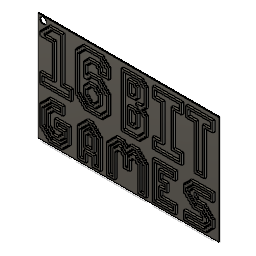
16 Bit Logo v8 (Autodesk Fusion 360 design; units mm, degrees)
Autodesk Fusion 360 part; units mm, degrees
(part 1 of 2)
sketch "Sketch1" plane through (0, 0, 0) normal (0, 0, 1) x (1, 0, 0)
  line L0 (0, 48) -> (4, 48)
  line L1 (4, 48) -> (4, 47)
  line L2 (4, 47) -> (3, 47)
  line L3 (3, 47) -> (3, 46)
  line L4 (3, 46) -> (2, 46)
  line L5 (2, 46) -> (2, 45)
  line L6 (2, 45) -> (1, 45)
  line L7 (1, 45) -> (1, 44)
  line L8 (1, 44) -> (0, 44)
  line L9 (0, 44) -> (0, 42)
  line L10 (0, 42) -> (6, 42)
  line L11 (6, 42) -> (6, 27)
  line L12 (6, 27) -> (0, 27)
  line L13 (0, 27) -> (0, 26.9)
  line L14 (0, 27) -> (0, 22)
  line L15 (7, 42) -> (7, 27)
  line L16 (7, 27) -> (7, 26)
  line L17 (7, 26) -> (1, 26)
  line L18 (0, 22) -> (15, 22)
  line L19 (15, 22) -> (15, 27)
  line L20 (15, 27) -> (11, 27)
  line L21 (11, 27) -> (11, 48)
  line L22 (1, 26) -> (1, 23)
  line L23 (1, 23) -> (14, 23)
  line L24 (14, 23) -> (14, 26)
  line L25 (14, 26) -> (10, 26)
  line L26 (10, 26) -> (10, 47)
  line L27 (10, 47) -> (5, 47)
  line L28 (5, 47) -> (5, 46)
  line L29 (5, 46) -> (4, 46)
  line L30 (4, 46) -> (4, 45)
  line L31 (4, 45) -> (3, 45)
  line L32 (3, 45) -> (3, 44)
  line L33 (3, 44) -> (2, 44)
  line L34 (2, 44) -> (2, 43)
  line L35 (2, 43) -> (6, 43)
  line L36 (7, 42) -> (7, 43)
  line L37 (7, 43) -> (6, 43)
  line L38 (17, 27) -> (17, 26)
  line L39 (17, 26) -> (18, 26)
  line L40 (18, 26) -> (18, 25)
  line L41 (18, 25) -> (19, 25)
  line L42 (19, 25) -> (19, 24)
  line L43 (19, 24) -> (20, 24)
  line L44 (20, 24) -> (20, 23)
  line L45 (20, 23) -> (21, 23)
  line L46 (21, 23) -> (21, 22)
  line L47 (21, 22) -> (30, 22)
  line L48 (30, 22) -> (30, 23)
  line L49 (30, 23) -> (31, 23)
  line L50 (31, 23) -> (31, 24)
  line L51 (31, 24) -> (32, 24)
  line L52 (32, 24) -> (32, 25)
  line L53 (32, 25) -> (33, 25)
  line L54 (33, 25) -> (33, 34)
  line L55 (33, 34) -> (32, 34)
  line L56 (32, 34) -> (32, 35)
  line L57 (32, 35) -> (31, 35)
  line L58 (31, 35) -> (31, 36)
  line L59 (31, 36) -> (30, 36)
  line L60 (30, 36) -> (30, 37)
  line L61 (30, 37) -> (29, 37)
  line L62 (29, 37) -> (29, 38)
  line L63 (29, 38) -> (23, 38)
  line L64 (23, 38) -> (23, 37)
  line L65 (23, 37) -> (22, 37)
  line L66 (22, 37) -> (22, 41)
  line L67 (22, 41) -> (23, 41)
  line L68 (23, 41) -> (23, 42)
  line L69 (23, 42) -> (24, 42)
  line L70 (24, 42) -> (24, 43)
  line L71 (24, 43) -> (27, 43)
  line L72 (27, 43) -> (27, 42)
  line L73 (27, 42) -> (28, 42)
  line L74 (28, 42) -> (28, 41)
  line L75 (28, 41) -> (28, 40)
  line L76 (28, 40) -> (33, 40)
  line L77 (33, 40) -> (33, 45)
  line L78 (33, 45) -> (32, 45)
  line L79 (32, 45) -> (32, 46)
  line L80 (32, 46) -> (31, 46)
  line L81 (31, 46) -> (31, 47)
  line L82 (31, 47) -> (30, 47)
  line L83 (30, 47) -> (30, 48)
  line L84 (17, 27) -> (17, 45)
  line L85 (17, 45) -> (18, 45)
  line L86 (18, 45) -> (18, 46)
  line L87 (18, 46) -> (19, 46)
  line L88 (19, 46) -> (19, 47)
  line L89 (19, 47) -> (20, 47)
  line L90 (20, 47) -> (20, 48)
  line L91 (29, 41) -> (32, 41)
  line L92 (32, 41) -> (32, 44)
  line L93 (32, 44) -> (31, 44)
  line L94 (31, 44) -> (31, 45)
  line L95 (31, 45) -> (30, 45)
  line L96 (30, 45) -> (30, 46)
  line L97 (30, 46) -> (29, 46)
  line L98 (29, 46) -> (29, 47)
  line L99 (29, 47) -> (21, 47)
  line L100 (21, 47) -> (21, 46)
  line L101 (21, 46) -> (20, 46)
  line L102 (20, 46) -> (20, 45)
  line L103 (20, 45) -> (19, 45)
  line L104 (19, 45) -> (19, 44)
  line L105 (19, 44) -> (18, 44)
  line L106 (18, 44) -> (18, 27)
  line L107 (18, 27) -> (19, 27)
  line L108 (19, 27) -> (19, 26)
  line L109 (19, 26) -> (20, 26)
  line L110 (20, 26) -> (20, 25)
  line L111 (20, 25) -> (21, 25)
  line L112 (21, 25) -> (21, 24)
  line L113 (21, 24) -> (22, 24)
  line L114 (22, 24) -> (22, 23)
  line L115 (22, 23) -> (29, 23)
  line L116 (29, 23) -> (29, 24)
  line L117 (29, 24) -> (29, 23)
  line L118 (29, 24) -> (30, 24)
  line L119 (30, 24) -> (30, 25)
  line L120 (30, 25) -> (31, 25)
  line L121 (31, 25) -> (31, 26)
  line L122 (31, 26) -> (32, 26)
  line L123 (32, 26) -> (32, 33)
  line L124 (32, 33) -> (31, 33)
  line L125 (31, 33) -> (31, 34)
  line L126 (31, 34) -> (30, 34)
  line L127 (30, 34) -> (30, 35)
  line L128 (30, 35) -> (29, 35)
  line L129 (29, 35) -> (30, 35)
  line L130 (29, 35) -> (29, 36)
  line L131 (29, 36) -> (28, 36)
  line L132 (28, 36) -> (28, 37)
  line L133 (28, 37) -> (24, 37)
  line L134 (24, 37) -> (24, 36)
  line L135 (24, 36) -> (23, 36)
  line L136 (23, 36) -> (23, 35)
  line L137 (23, 35) -> (21, 35)
  line L138 (21, 35) -> (21, 42)
  line L139 (21, 42) -> (22, 42)
  line L140 (22, 42) -> (22, 43)
  line L141 (22, 43) -> (23, 43)
  line L142 (23, 43) -> (23, 44)
  line L143 (23, 44) -> (28, 44)
  line L144 (28, 44) -> (28, 43)
  line L145 (28, 43) -> (29, 43)
  line L146 (29, 41) -> (29, 43)
  line L147 (23, 34) -> (27, 34)
  line L148 (27, 34) -> (27, 33)
  line L149 (27, 33) -> (28, 33)
  line L150 (28, 33) -> (28, 32)
  line L151 (28, 32) -> (29, 32)
  line L152 (29, 32) -> (28, 32)
  line L153 (29, 32) -> (29, 27)
  line L154 (29, 27) -> (28, 27)
  line L155 (28, 27) -> (28, 26)
  line L156 (28, 26) -> (27, 26)
  line L157 (27, 26) -> (27, 25)
  line L158 (27, 25) -> (23, 25)
  line L159 (23, 25) -> (23, 26)
  line L160 (23, 26) -> (23, 25)
  line L161 (23, 26) -> (22, 26)
  line L162 (22, 26) -> (22, 27)
  line L163 (22, 27) -> (21, 27)
  line L164 (21, 27) -> (21, 32)
  line L165 (21, 32) -> (22, 32)
  line L166 (22, 32) -> (22, 33)
  line L167 (22, 33) -> (23, 33)
  line L168 (23, 33) -> (23, 34)
  line L169 (23, 32) -> (24, 32)
  line L170 (24, 32) -> (24, 33)
  line L171 (24, 33) -> (26, 33)
  line L172 (26, 33) -> (26, 32)
  line L173 (26, 32) -> (27, 32)
  line L174 (27, 32) -> (27, 31)
  line L175 (27, 31) -> (28, 31)
  line L176 (28, 31) -> (28, 28)
  line L177 (28, 28) -> (27, 28)
  line L178 (27, 28) -> (27, 27)
  line L179 (27, 27) -> (26, 27)
  line L180 (26, 27) -> (26, 26)
  line L181 (24, 26) -> (26, 26)
  line L182 (24, 26) -> (24, 27)
  line L183 (24, 27) -> (23, 27)
  line L184 (23, 27) -> (23, 28)
  line L185 (23, 28) -> (22, 28)
  line L186 (22, 28) -> (22, 31)
  line L187 (22, 31) -> (23, 31)
  line L188 (23, 31) -> (22, 31)
  line L189 (23, 31) -> (23, 32)
  line L190 (30, 48) -> (39, 48)
  line L191 (39, 48) -> (39, 22)
  line L192 (39, 22) -> (48, 22)
  line L193 (48, 22) -> (48, 23)
  line L194 (48, 23) -> (49, 23)
  line L195 (49, 23) -> (49, 24)
  line L196 (49, 24) -> (50, 24)
  line L197 (50, 24) -> (50, 25)
  line L198 (50, 25) -> (51, 25)
  line L199 (51, 25) -> (51, 34)
  line L200 (51, 34) -> (50, 34)
  line L201 (50, 34) -> (50, 35)
  line L202 (50, 35) -> (49, 35)
  line L203 (49, 35) -> (49, 36)
  line L204 (49, 36) -> (50, 36)
  line L205 (50, 36) -> (50, 37)
  line L206 (50, 37) -> (51, 37)
  line L207 (51, 37) -> (51, 46)
  line L208 (51, 46) -> (50, 46)
  line L209 (50, 46) -> (50, 47)
  line L210 (50, 47) -> (49, 47)
  line L211 (49, 47) -> (49, 48)
  line L212 (40, 23) -> (40, 47)
  line L213 (40, 47) -> (48, 47)
  line L214 (48, 47) -> (48, 46)
  line L215 (48, 46) -> (49, 46)
  line L216 (49, 46) -> (49, 45)
  line L217 (49, 45) -> (50, 45)
  line L218 (50, 45) -> (50, 38)
  line L219 (50, 38) -> (49, 38)
  line L220 (49, 38) -> (49, 37)
  line L221 (49, 37) -> (46, 37)
  line L222 (46, 37) -> (46, 36)
  line L223 (46, 36) -> (47, 36)
  line L224 (47, 36) -> (47, 35)
  line L225 (47, 35) -> (48, 35)
  line L226 (48, 35) -> (48, 34)
  line L227 (48, 34) -> (49, 34)
  line L228 (49, 34) -> (49, 33)
  line L229 (49, 33) -> (50, 33)
  line L230 (50, 26) -> (50, 33)
  line L231 (50, 26) -> (49, 26)
  line L232 (49, 26) -> (49, 25)
  line L233 (49, 25) -> (48, 25)
  line L234 (48, 25) -> (48, 24)
  line L235 (48, 24) -> (47, 24)
  line L236 (47, 24) -> (47, 23)
  line L237 (47, 23) -> (40, 23)
  line L238 (46, 26) -> (46, 27)
  line L239 (46, 27) -> (47, 27)
  line L240 (47, 27) -> (47, 33)
  line L241 (47, 33) -> (46, 33)
  line L242 (46, 33) -> (46, 34)
  line L243 (46, 34) -> (42, 34)
  line L244 (42, 34) -> (42, 26)
  line L245 (42, 26) -> (46, 26)
  line L246 (43, 27) -> (43, 33)
  line L247 (43, 33) -> (45, 33)
  line L248 (45, 33) -> (45, 32)
  line L249 (45, 32) -> (46, 32)
  line L250 (46, 32) -> (46, 28)
  line L251 (46, 28) -> (45, 28)
  line L252 (45, 28) -> (45, 27)
  line L253 (43, 27) -> (45, 27)
  line L254 (42, 39) -> (42, 45)
  line L255 (42, 45) -> (46, 45)
  line L256 (46, 45) -> (46, 44)
  line L257 (46, 44) -> (47, 44)
  line L258 (47, 44) -> (47, 39)
  line L259 (47, 39) -> (46, 39)
  line L260 (46, 39) -> (46, 38)
  line L261 (46, 38) -> (42, 38)
  line L262 (42, 38) -> (42, 39)
  line L263 (43, 39) -> (43, 44)
  line L264 (45, 44) -> (43, 44)
  line L265 (45, 44) -> (45, 43)
  line L266 (45, 43) -> (46, 43)
  line L267 (46, 43) -> (46, 40)
  line L268 (46, 40) -> (45, 40)
  line L269 (45, 40) -> (45, 39)
  line L270 (43, 39) -> (45, 39)
  line L271 (49, 48) -> (54, 48)
  line L272 (54, 48) -> (54, 43)
  line L273 (54, 22) -> (54, 27)
  line L274 (54, 27) -> (58, 27)
  line L275 (58, 27) -> (58, 43)
  line L276 (58, 43) -> (54, 43)
  line L277 (54, 22) -> (68, 22)
  line L278 (68, 22) -> (68, 27)
  line L279 (68, 27) -> (64, 27)
  line L280 (64, 27) -> (64, 43)
  line L281 (64, 43) -> (68, 43)
  line L282 (68, 43) -> (68, 48)
  line L283 (55, 47) -> (55, 44)
  line L284 (55, 44) -> (59, 44)
  line L285 (59, 44) -> (59, 26)
  line L286 (59, 26) -> (55, 26)
  line L287 (55, 26) -> (55, 23)
  line L288 (55, 23) -> (67, 23)
  line L289 (67, 23) -> (67, 26)
  line L290 (67, 26) -> (63, 26)
  line L291 (63, 26) -> (63, 44)
  line L292 (63, 44) -> (67, 44)
  line L293 (67, 44) -> (67, 47)
  line L294 (67, 47) -> (55, 47)
  line L295 (70, 43) -> (70, 48)
  line L296 (70, 43) -> (74, 43)
  line L297 (74, 43) -> (74, 22)
  line L298 (74, 22) -> (79, 22)
  line L299 (79, 22) -> (79, 43)
  line L300 (79, 43) -> (82, 43)
  line L301 (82, 43) -> (83, 43)
  line L302 (83, 43) -> (83, 48)
  line L303 (83, 48) -> (82, 48)
  line L304 (71, 47) -> (82, 47)
  line L305 (82, 47) -> (82, 44)
  line L306 (82, 44) -> (78, 44)
  line L307 (78, 44) -> (78, 23)
  line L308 (78, 23) -> (75, 23)
  line L309 (75, 23) -> (78, 23)
  line L310 (75, 23) -> (75, 44)
  line L311 (75, 44) -> (71, 44)
  line L312 (71, 44) -> (71, 47)
  line L313 (0, 0) -> (83, 0)
  line L314 (83, 0) -> (83, 48)
  line L315 (83, 48) -> (0, 48)
  line L316 (0, 48) -> (0, 0)
  line L317 (0, 0) -> (0, 1)
  line L318 (0, 0) -> (0, 4)
  line L319 (0, 4) -> (1, 4)
  line L320 (1, 4) -> (1, 3)
  line L321 (1, 3) -> (2, 3)
  line L322 (2, 3) -> (2, 2)
  line L323 (2, 2) -> (3, 2)
  line L324 (3, 2) -> (3, 1)
  line L325 (3, 1) -> (4, 1)
  line L326 (4, 1) -> (4, 0)
  line L327 (4, 0) -> (11, 0)
  line L328 (4, 0) -> (11, 0)
  line L329 (11, 0) -> (11, 1)
  line L330 (11, 1) -> (12, 1)
  line L331 (12, 1) -> (12, 2)
  line L332 (12, 2) -> (13, 2)
  line L333 (13, 2) -> (13, 3)
  line L334 (13, 3) -> (14, 3)
  line L335 (14, 3) -> (14, 11)
  line L336 (14, 11) -> (7, 11)
  line L337 (7, 11) -> (7, 7)
  line L338 (7, 7) -> (11, 7)
  line L339 (11, 7) -> (11, 6)
  line L340 (11, 6) -> (10, 6)
  line L341 (10, 6) -> (10, 5)
  line L342 (10, 5) -> (9, 5)
  line L343 (9, 5) -> (9, 4)
  line L344 (9, 4) -> (6, 4)
  line L345 (6, 4) -> (6, 5)
  line L346 (6, 5) -> (5, 5)
  line L347 (5, 5) -> (5, 6)
  line L348 (5, 6) -> (4, 6)
  line L349 (4, 6) -> (4, 12)
  line L350 (4, 12) -> (5, 12)
  line L351 (5, 12) -> (5, 13)
  line L352 (5, 13) -> (6, 13)
  line L353 (6, 13) -> (6, 14)
  line L354 (6, 14) -> (11, 14)
  line L355 (11, 14) -> (11, 18)
  line L356 (11, 18) -> (4, 18)
  line L357 (4, 18) -> (4, 17)
  line L358 (4, 17) -> (3, 17)
  line L359 (3, 17) -> (3, 16)
  line L360 (3, 16) -> (2, 16)
  line L361 (2, 16) -> (2, 15)
  line L362 (2, 15) -> (1, 15)
  line L363 (1, 15) -> (1, 14)
  line L364 (1, 14) -> (0, 14)
  line L365 (1, 13) -> (1, 5)
  line L366 (1, 5) -> (2, 5)
  line L367 (2, 5) -> (2, 4)
  line L368 (2, 4) -> (3, 4)
  line L369 (3, 4) -> (3, 3)
  line L370 (3, 3) -> (4, 3)
  line L371 (4, 3) -> (4, 2)
  line L372 (4, 2) -> (5, 2)
  line L373 (5, 2) -> (5, 1)
  line L374 (5, 1) -> (10, 1)
  line L375 (10, 1) -> (10, 2)
  line L376 (10, 2) -> (11, 2)
  line L377 (11, 2) -> (11, 3)
  line L378 (11, 3) -> (12, 3)
  line L379 (12, 3) -> (12, 4)
  line L380 (12, 4) -> (13, 4)
  line L381 (13, 4) -> (13, 10)
  line L382 (13, 10) -> (8, 10)
  line L383 (8, 10) -> (8, 8)
  line L384 (8, 8) -> (12, 8)
  line L385 (12, 8) -> (12, 5)
  line L386 (12, 5) -> (11, 5)
  line L387 (11, 5) -> (11, 4)
  line L388 (11, 4) -> (10, 4)
  line L389 (10, 4) -> (10, 3)
  line L390 (10, 3) -> (5, 3)
  line L391 (5, 3) -> (5, 4)
  line L392 (5, 4) -> (4, 4)
  line L393 (4, 4) -> (4, 5)
  line L394 (4, 5) -> (3, 5)
  line L395 (3, 5) -> (3, 13)
  line L396 (3, 13) -> (4, 13)
  line L397 (4, 13) -> (4, 14)
  line L398 (4, 14) -> (5, 14)
  line L399 (5, 14) -> (5, 15)
  line L400 (5, 15) -> (10, 15)
  line L401 (10, 15) -> (10, 17)
  line L402 (10, 17) -> (5, 17)
  line L403 (5, 17) -> (5, 16)
  line L404 (5, 16) -> (4, 16)
  line L405 (4, 16) -> (4, 15)
  line L406 (4, 15) -> (3, 15)
  line L407 (3, 15) -> (3, 14)
  line L408 (3, 14) -> (2, 14)
  line L409 (2, 14) -> (2, 13)
  line L410 (2, 13) -> (1, 13)
  line L411 (11, 0) -> (12, 0)
  line L412 (11, 0) -> (18, 0)
  line L413 (18, 0) -> (18, 14)
  line L414 (18, 14) -> (19, 14)
  line L415 (19, 14) -> (19, 15)
  line L416 (19, 15) -> (20, 15)
  line L417 (20, 15) -> (20, 16)
  line L418 (20, 16) -> (21, 16)
  line L419 (21, 16) -> (21, 17)
  line L420 (21, 17) -> (22, 17)
  line L421 (22, 17) -> (22, 18)
  line L422 (22, 18) -> (25, 18)
  line L423 (25, 18) -> (25, 17)
  line L424 (25, 17) -> (26, 17)
  line L425 (26, 17) -> (26, 16)
  line L426 (26, 16) -> (27, 16)
  line L427 (27, 16) -> (27, 15)
  line L428 (27, 15) -> (28, 15)
  line L429 (28, 15) -> (28, 14)
  line L430 (28, 14) -> (29, 14)
  line L431 (29, 14) -> (29, 0)
  line L432 (28, 1) -> (28, 13)
  line L433 (28, 13) -> (27, 13)
  line L434 (27, 13) -> (27, 14)
  line L435 (27, 14) -> (26, 14)
  line L436 (26, 14) -> (26, 15)
  line L437 (26, 15) -> (25, 15)
  line L438 (25, 15) -> (25, 16)
  line L439 (25, 16) -> (24, 16)
  line L440 (24, 16) -> (24, 17)
  line L441 (24, 17) -> (23, 17)
  line L442 (23, 17) -> (23, 16)
  line L443 (23, 16) -> (22, 16)
  line L444 (22, 16) -> (22, 15)
  line L445 (22, 15) -> (21, 15)
  line L446 (21, 15) -> (21, 14)
  line L447 (21, 14) -> (20, 14)
  line L448 (20, 14) -> (20, 13)
  line L449 (20, 13) -> (19, 13)
  line L450 (28, 1) -> (26, 1)
  line L451 (19, 1) -> (21, 1)
  line L452 (19, 13) -> (19, 1)
  line L453 (22, 0) -> (22, 4)
  line L454 (22, 4) -> (25, 4)
  line L455 (25, 4) -> (25, 0)
  line L456 (25, 5) -> (22, 5)
  line L457 (22, 5) -> (21, 5)
  line L458 (25, 5) -> (26, 5)
  line L459 (26, 1) -> (26, 5)
  line L460 (21, 5) -> (21, 1)
  line L461 (21, 6) -> (26, 6)
  line L462 (26, 6) -> (26, 13)
  line L463 (26, 13) -> (25, 13)
  line L464 (25, 13) -> (25, 14)
  line L465 (25, 14) -> (24, 14)
  line L466 (24, 14) -> (24, 15)
  line L467 (24, 15) -> (23, 15)
  line L468 (23, 15) -> (23, 14)
  line L469 (23, 14) -> (22, 14)
  line L470 (22, 14) -> (22, 13)
  line L471 (22, 13) -> (21, 13)
  line L472 (21, 13) -> (21, 6)
  line L473 (29, 0) -> (32, 0)
  line L474 (32, 0) -> (32, 14)
  line L475 (32, 14) -> (33, 14)
  line L476 (33, 14) -> (33, 15)
  line L477 (33, 15) -> (34, 15)
  line L478 (34, 15) -> (34, 16)
  line L479 (34, 16) -> (35, 16)
  line L480 (35, 16) -> (35, 17)
  line L481 (35, 17) -> (36, 17)
  line L482 (36, 17) -> (36, 18)
  line L483 (36, 18) -> (40, 18)
  line L484 (40, 18) -> (40, 17)
  line L485 (40, 17) -> (41, 17)
  line L486 (41, 17) -> (41, 16)
  line L487 (41, 16) -> (42, 16)
  line L488 (42, 16) -> (42, 17)
  line L489 (42, 17) -> (43, 17)
  line L490 (43, 17) -> (43, 18)
  line L491 (43, 18) -> (47, 18)
  line L492 (47, 18) -> (47, 17)
  line L493 (47, 17) -> (48, 17)
  line L494 (48, 17) -> (48, 16)
  line L495 (48, 16) -> (49, 16)
  line L496 (49, 16) -> (49, 15)
  line L497 (49, 15) -> (50, 15)
  line L498 (50, 15) -> (50, 14)
  line L499 (50, 14) -> (51, 14)
  line L500 (51, 14) -> (51, 0)
  line L501 (50, 1) -> (50, 13)
  line L502 (50, 13) -> (49, 13)
  line L503 (49, 13) -> (49, 14)
  line L504 (49, 14) -> (48, 14)
  line L505 (48, 14) -> (48, 15)
  line L506 (48, 15) -> (47, 15)
  line L507 (47, 15) -> (47, 16)
  line L508 (47, 16) -> (46, 16)
  line L509 (46, 16) -> (46, 17)
  line L510 (46, 17) -> (44, 17)
  line L511 (44, 17) -> (44, 16)
  line L512 (44, 16) -> (43, 16)
  line L513 (43, 16) -> (43, 15)
  line L514 (43, 15) -> (42, 15)
  line L515 (42, 15) -> (42, 14)
  line L516 (42, 14) -> (41, 14)
  line L517 (41, 14) -> (41, 15)
  line L518 (41, 15) -> (40, 15)
  line L519 (40, 15) -> (40, 16)
  line L520 (40, 16) -> (39, 16)
  line L521 (39, 16) -> (39, 17)
  line L522 (39, 17) -> (37, 17)
  line L523 (37, 17) -> (37, 16)
  line L524 (37, 16) -> (36, 16)
  line L525 (36, 16) -> (36, 15)
  line L526 (36, 15) -> (35, 15)
  line L527 (35, 15) -> (35, 14)
  line L528 (35, 14) -> (34, 14)
  line L529 (34, 14) -> (34, 13)
  line L530 (34, 13) -> (33, 13)
  line L531 (33, 13) -> (33, 1)
  line L532 (33, 1) -> (35, 1)
  line L533 (35, 1) -> (35, 13)
  line L534 (35, 13) -> (36, 13)
  line L535 (36, 13) -> (36, 14)
  line L536 (36, 14) -> (37, 14)
  line L537 (37, 14) -> (37, 15)
  line L538 (37, 15) -> (39, 15)
  line L539 (39, 15) -> (39, 14)
  line L540 (39, 14) -> (40, 14)
  line L541 (40, 14) -> (40, 13)
  line L542 (40, 13) -> (41, 13)
  line L543 (41, 13) -> (41, 8)
  line L544 (41, 8) -> (42, 8)
  line L545 (42, 8) -> (42, 13)
  line L546 (42, 13) -> (43, 13)
  line L547 (43, 13) -> (43, 14)
  line L548 (43, 14) -> (44, 14)
  line L549 (44, 14) -> (44, 15)
  line L550 (44, 15) -> (46, 15)
  line L551 (46, 15) -> (46, 14)
  line L552 (46, 14) -> (47, 14)
  line L553 (47, 14) -> (47, 13)
  line L554 (47, 13) -> (48, 13)
  line L555 (48, 13) -> (48, 1)
  line L556 (48, 1) -> (50, 1)
  line L557 (47, 0) -> (47, 12)
  line L558 (47, 12) -> (46, 12)
  line L559 (46, 12) -> (46, 13)
  line L560 (46, 13) -> (44, 13)
  line L561 (44, 13) -> (44, 12)
  line L562 (44, 12) -> (43, 12)
  line L563 (43, 12) -> (43, 7)
  line L564 (43, 7) -> (40, 7)
  line L565 (40, 7) -> (40, 12)
  line L566 (40, 12) -> (39, 12)
  line L567 (39, 12) -> (39, 13)
  line L568 (39, 13) -> (37, 13)
  line L569 (37, 13) -> (37, 12)
  line L570 (37, 12) -> (36, 12)
  line L571 (36, 12) -> (36, 0)
  line L572 (51, 0) -> (54, 0)
  line L573 (54, 0) -> (54, 18)
  line L574 (54, 18) -> (65, 18)
  line L575 (65, 18) -> (65, 14)
  line L576 (65, 14) -> (58, 14)
  line L577 (58, 14) -> (58, 11)
  line L578 (58, 11) -> (61, 11)
  line L579 (61, 11) -> (61, 7)
  line L580 (61, 7) -> (58, 7)
  line L581 (58, 7) -> (58, 4)
  line L582 (58, 4) -> (65, 4)
  line L583 (65, 4) -> (65, 0)
  line L584 (64, 1) -> (64, 3)
  line L585 (64, 3) -> (57, 3)
  line L586 (57, 3) -> (57, 8)
  line L587 (57, 8) -> (60, 8)
  line L588 (60, 8) -> (60, 10)
  line L589 (60, 10) -> (57, 10)
  line L590 (57, 10) -> (57, 15)
  line L591 (57, 15) -> (64, 15)
  line L592 (64, 15) -> (64, 17)
  line L593 (64, 17) -> (55, 17)
  line L594 (55, 17) -> (55, 1)
  line L595 (55, 1) -> (64, 1)
  line L596 (65, 0) -> (69, 0)
  line L597 (69, 4) -> (69, 0)
  line L598 (69, 4) -> (78, 4)
  line L599 (78, 4) -> (78, 6)
  line L600 (78, 6) -> (77, 6)
  line L601 (77, 6) -> (77, 7)
  line L602 (77, 7) -> (73, 7)
  line L603 (73, 7) -> (73, 8)
  line L604 (73, 8) -> (72, 8)
  line L605 (72, 8) -> (72, 9)
  line L606 (72, 9) -> (71, 9)
  line L607 (71, 9) -> (71, 10)
  line L608 (71, 10) -> (70, 10)
  line L609 (70, 10) -> (70, 11)
  line L610 (70, 11) -> (69, 11)
  line L611 (69, 11) -> (69, 15)
  line L612 (69, 15) -> (70, 15)
  line L613 (70, 15) -> (70, 16)
  line L614 (70, 16) -> (71, 16)
  line L615 (71, 16) -> (71, 17)
  line L616 (71, 17) -> (72, 17)
  line L617 (72, 17) -> (72, 18)
  line L618 (83, 18) -> (83, 14)
  line L619 (83, 18) -> (72, 18)
  line L620 (83, 14) -> (74, 14)
  line L621 (74, 14) -> (74, 12)
  line L622 (74, 12) -> (75, 12)
  line L623 (75, 12) -> (75, 11)
  line L624 (75, 11) -> (79, 11)
  line L625 (79, 11) -> (79, 10)
  line L626 (79, 10) -> (80, 10)
  line L627 (80, 10) -> (80, 9)
  line L628 (80, 9) -> (81, 9)
  line L629 (81, 9) -> (81, 8)
  line L630 (81, 8) -> (82, 8)
  line L631 (82, 8) -> (82, 7)
  line L632 (82, 7) -> (83, 7)
  line L633 (83, 7) -> (83, 3)
  line L634 (83, 3) -> (82, 3)
  line L635 (82, 3) -> (82, 2)
  line L636 (82, 2) -> (81, 2)
  line L637 (81, 2) -> (81, 1)
  line L638 (81, 1) -> (80, 1)
  line L639 (80, 1) -> (80, 0)
  line L640 (70, 1) -> (79, 1)
  line L641 (79, 1) -> (79, 2)
  line L642 (79, 2) -> (80, 2)
  line L643 (80, 2) -> (80, 3)
  line L644 (80, 3) -> (81, 3)
  line L645 (81, 3) -> (81, 4)
  line L646 (81, 4) -> (82, 4)
  line L647 (82, 4) -> (82, 6)
  line L648 (82, 6) -> (81, 6)
  line L649 (81, 6) -> (81, 7)
  line L650 (81, 7) -> (80, 7)
  line L651 (80, 7) -> (80, 8)
  line L652 (80, 8) -> (79, 8)
  line L653 (79, 8) -> (79, 9)
  line L654 (79, 9) -> (78, 9)
  line L655 (78, 9) -> (78, 10)
  line L656 (78, 10) -> (74, 10)
  line L657 (74, 10) -> (74, 11)
  line L658 (74, 11) -> (73, 11)
  line L659 (73, 11) -> (73, 12)
  line L660 (73, 12) -> (72, 12)
  line L661 (82, 15) -> (82, 17)
  line L662 (82, 17) -> (73, 17)
  line L663 (73, 17) -> (73, 16)
  line L664 (73, 16) -> (72, 16)
  line L665 (72, 16) -> (72, 15)
  line L666 (72, 14) -> (73, 14)
  line L667 (73, 14) -> (73, 15)
  line L668 (72, 14) -> (72, 12)
  line L669 (73, 15) -> (82, 15)
  line L670 (72, 15) -> (71, 15)
  line L671 (71, 15) -> (71, 14)
  line L672 (71, 14) -> (70, 14)
  line L673 (70, 14) -> (70, 12)
  line L674 (70, 12) -> (71, 12)
  line L675 (71, 12) -> (71, 11)
  line L676 (71, 11) -> (72, 11)
  line L677 (72, 11) -> (72, 10)
  line L678 (72, 10) -> (73, 10)
  line L679 (73, 10) -> (73, 9)
  line L680 (73, 9) -> (74, 9)
  line L681 (74, 9) -> (74, 8)
  line L682 (74, 8) -> (78, 8)
  line L683 (78, 8) -> (78, 7)
  line L684 (78, 7) -> (79, 7)
  line L685 (79, 7) -> (79, 6)
  line L686 (79, 6) -> (80, 6)
  line L687 (80, 6) -> (80, 4)
  line L688 (80, 4) -> (79, 4)
  line L689 (79, 4) -> (79, 3)
  line L690 (79, 3) -> (70, 3)
  line L691 (70, 3) -> (70, 1)
  line L692 (22, 7) -> (22, 12)
  line L693 (22, 12) -> (23, 12)
  line L694 (23, 12) -> (23, 13)
  line L695 (23, 13) -> (24, 13)
  line L696 (24, 13) -> (24, 12)
  line L697 (24, 12) -> (25, 12)
  line L698 (-1, -1) -> (84, -1)
  line L699 (84, -1) -> (84, 49)
  line L700 (84, 49) -> (-1, 49)
  line L701 (-1, 49) -> (-1, -1)
  line L702 (25, 12) -> (25, 7)
  line L703 (25, 7) -> (22, 7)
  dimension "d3" = 4
  dimension "d4" = 1
  dimension "d5" = 1
  dimension "d6" = 1
  dimension "d7" = 1
  dimension "d8" = 1
  dimension "d9" = 1
  dimension "d10" = 1
  dimension "d11" = 2
  dimension "d12" = 6
  dimension "d13" = 15
  dimension "d14" = 5
  dimension "d18" = 1
  dimension "d19" = 6
  dimension "d20" = 15
  dimension "d21" = 5
  dimension "d22" = 4
  dimension "d23" = 3
  dimension "d24" = 5
  constraint perpendicular L1 L2
  constraint perpendicular L2 L3
  constraint perpendicular L3 L4
  constraint perpendicular L4 L5
  constraint perpendicular L5 L6
  constraint perpendicular L6 L7
  constraint perpendicular L8 L9
  constraint perpendicular L10 L11
  constraint perpendicular L12 L14
  constraint perpendicular L14 L17
  constraint perpendicular L18 L19
  constraint perpendicular L19 L20
  constraint perpendicular L17 L22
  constraint perpendicular L22 L23
  constraint perpendicular L23 L24
  constraint perpendicular L24 L25
  constraint perpendicular L23 L26
  constraint perpendicular L26 L27
  constraint perpendicular L27 L28
  constraint perpendicular L28 L29
  constraint perpendicular L29 L30
  constraint perpendicular L30 L31
  constraint perpendicular L31 L32
  constraint perpendicular L32 L33
  constraint perpendicular L33 L34
  constraint perpendicular L34 L35
  constraint parallel L15 L36
  constraint perpendicular L18 L38
  constraint perpendicular L38 L39
  constraint perpendicular L39 L40
  constraint perpendicular L40 L41
  constraint perpendicular L41 L42
  constraint perpendicular L42 L43
  constraint perpendicular L43 L44
  constraint perpendicular L44 L45
  constraint perpendicular L45 L46
  constraint perpendicular L46 L47
  constraint perpendicular L45 L48
  constraint perpendicular L48 L49
  constraint perpendicular L49 L50
  constraint perpendicular L50 L51
  constraint perpendicular L51 L52
  constraint perpendicular L52 L53
  constraint perpendicular L53 L54
  constraint perpendicular L54 L55
  constraint perpendicular L23 L56
  constraint perpendicular L56 L57
  constraint perpendicular L57 L58
  constraint perpendicular L58 L59
  constraint perpendicular L59 L60
  constraint perpendicular L60 L61
  constraint perpendicular L61 L62
  constraint perpendicular L62 L63
  constraint perpendicular L63 L64
  constraint perpendicular L62 L65
  constraint perpendicular L65 L66
  constraint perpendicular L66 L67
  constraint perpendicular L67 L68
  constraint perpendicular L66 L69
  constraint perpendicular L69 L70
  constraint perpendicular L66 L71
  constraint perpendicular L71 L72
  constraint perpendicular L72 L73
  constraint perpendicular L73 L74
  constraint perpendicular L23 L75
  constraint perpendicular L75 L76
  constraint perpendicular L73 L77
  constraint perpendicular L77 L78
  constraint perpendicular L73 L79
  constraint perpendicular L79 L80
  constraint perpendicular L73 L81
  constraint perpendicular L81 L82
  constraint perpendicular L84 L85
  constraint perpendicular L86 L87
  constraint perpendicular L87 L88
  constraint perpendicular L88 L89
  constraint perpendicular L77 L91
  constraint perpendicular L92 L93
  constraint perpendicular L93 L94
  constraint perpendicular L94 L95
  constraint perpendicular L95 L96
  constraint perpendicular L96 L97
  constraint perpendicular L97 L98
  constraint perpendicular L96 L99
  constraint perpendicular L97 L100
  constraint perpendicular L96 L101
  constraint perpendicular L97 L102
  constraint perpendicular L102 L103
  constraint perpendicular L103 L104
  constraint perpendicular L102 L105
  constraint perpendicular L103 L106
  constraint perpendicular L102 L107
  constraint perpendicular L103 L108
  constraint perpendicular L102 L109
  constraint perpendicular L103 L110
  constraint perpendicular L102 L111
  constraint perpendicular L103 L112
  constraint perpendicular L102 L113
  constraint perpendicular L113 L114
  constraint perpendicular L102 L115
  constraint perpendicular L113 L116
  constraint perpendicular L117 L118
  constraint perpendicular L115 L119
  constraint perpendicular L117 L120
  constraint perpendicular L115 L121
  constraint perpendicular L117 L122
  constraint perpendicular L115 L123
  constraint perpendicular L117 L124
  constraint perpendicular L115 L125
  constraint perpendicular L125 L126
  constraint perpendicular L115 L127
  constraint perpendicular L125 L128
  constraint perpendicular L128 L130
  constraint perpendicular L130 L131
  constraint perpendicular L128 L132
  constraint perpendicular L132 L133
  constraint perpendicular L128 L134
  constraint perpendicular L56 L135
  constraint perpendicular L57 L136
  constraint perpendicular L136 L137
  constraint perpendicular L137 L138
  constraint perpendicular L136 L139
  constraint perpendicular L139 L140
  constraint perpendicular L140 L141
  constraint perpendicular L141 L142
  constraint perpendicular L142 L143
  constraint perpendicular L143 L144
  constraint perpendicular L142 L145
  constraint perpendicular L91 L146
  constraint perpendicular L19 L147
  constraint perpendicular L19 L149
  constraint perpendicular L113 L150
  constraint perpendicular L112 L151
  constraint perpendicular L152 L153
  constraint perpendicular L58 L154
  constraint perpendicular L152 L155
  constraint perpendicular L155 L156
  constraint perpendicular L156 L157
  constraint perpendicular L157 L158
  constraint perpendicular L156 L159
  constraint perpendicular L160 L161
  constraint perpendicular L158 L162
  constraint perpendicular L160 L163
  constraint perpendicular L147 L164
  constraint perpendicular L147 L166
  constraint perpendicular L166 L167
  constraint perpendicular L147 L168
  constraint perpendicular L168 L169
  constraint perpendicular L167 L170
  constraint perpendicular L170 L171
  constraint perpendicular L171 L172
  constraint perpendicular L172 L173
  constraint perpendicular L173 L174
  constraint perpendicular L174 L175
  constraint perpendicular L173 L176
  constraint perpendicular L176 L177
  constraint perpendicular L173 L178
  constraint perpendicular L176 L179
  constraint perpendicular L173 L180
  constraint perpendicular L180 L181
  constraint perpendicular L181 L182
  constraint perpendicular L180 L183
  constraint perpendicular L181 L184
  constraint perpendicular L184 L185
  constraint perpendicular L185 L186
  constraint perpendicular L186 L187
  constraint perpendicular L169 L189
  constraint perpendicular L47 L191
  constraint perpendicular L191 L192
  constraint perpendicular L192 L193
  constraint perpendicular L191 L194
  constraint perpendicular L192 L195
  constraint perpendicular L191 L196
  constraint perpendicular L192 L197
  constraint perpendicular L191 L198
  constraint perpendicular L192 L199
  constraint perpendicular L191 L200
  constraint perpendicular L192 L201
  constraint perpendicular L191 L202
  constraint perpendicular L192 L203
  constraint perpendicular L203 L204
  constraint perpendicular L192 L205
  constraint perpendicular L203 L206
  constraint perpendicular L192 L207
  constraint perpendicular L207 L208
  constraint perpendicular L192 L209
  constraint perpendicular L207 L210
  constraint perpendicular L192 L212
  constraint perpendicular L191 L213
  constraint perpendicular L192 L214
  constraint perpendicular L214 L215
  constraint perpendicular L213 L216
  constraint perpendicular L214 L217
  constraint perpendicular L213 L218
  constraint perpendicular L214 L219
  constraint perpendicular L213 L220
  constraint perpendicular L220 L221
  constraint perpendicular L221 L222
  constraint perpendicular L220 L223
  constraint perpendicular L223 L224
  constraint perpendicular L224 L225
  constraint perpendicular L223 L226
  constraint perpendicular L224 L227
  constraint perpendicular L223 L228
  constraint perpendicular L228 L229
  constraint perpendicular L229 L230
  constraint perpendicular L230 L231
  constraint perpendicular L229 L232
  constraint perpendicular L230 L233
  constraint perpendicular L229 L234
  constraint perpendicular L230 L235
  constraint perpendicular L229 L236
  constraint perpendicular L212 L237
  constraint perpendicular L231 L238
  constraint perpendicular L199 L239
  constraint perpendicular L239 L240
  constraint perpendicular L238 L241
  constraint perpendicular L239 L242
  constraint perpendicular L191 L243
  constraint perpendicular L239 L244
  constraint perpendicular L238 L245
  constraint parallel L240 L246
  constraint perpendicular L246 L247
  constraint perpendicular L247 L248
  constraint perpendicular L248 L249
  constraint perpendicular L247 L250
  constraint perpendicular L248 L251
  constraint perpendicular L251 L252
  constraint perpendicular L252 L253
  constraint perpendicular L243 L254
  constraint perpendicular L223 L256
  constraint perpendicular L242 L257
  constraint perpendicular L122 L258
  constraint perpendicular L218 L259
  constraint perpendicular L122 L260
  constraint perpendicular L261 L262
  constraint vertical L263
  constraint coincident L263 L264.end
  constraint perpendicular L263 L264
  constraint perpendicular L264 L265
  constraint perpendicular L265 L266
  constraint perpendicular L266 L267
  constraint perpendicular L267 L268
  constraint perpendicular L268 L269
  constraint perpendicular L269 L270
  constraint perpendicular L211 L271
  constraint perpendicular L271 L272
  constraint perpendicular L192 L273
  constraint perpendicular L193 L274
  constraint perpendicular L192 L275
  constraint perpendicular L272 L276
  constraint perpendicular L273 L277
  constraint perpendicular L277 L278
  constraint perpendicular L273 L279
  constraint perpendicular L279 L280
  constraint perpendicular L280 L281
  constraint perpendicular L272 L284
  constraint perpendicular L284 L285
  constraint perpendicular L272 L286
  constraint perpendicular L284 L287
  constraint perpendicular L272 L288
  constraint perpendicular L284 L289
  constraint perpendicular L272 L290
  constraint perpendicular L284 L291
  constraint perpendicular L272 L292
  constraint perpendicular L284 L293
  constraint perpendicular L283 L294
  constraint perpendicular L295 L296
  constraint perpendicular L295 L298
  constraint perpendicular L300 L302
  constraint perpendicular L302 L304
  constraint perpendicular L304 L305
  constraint perpendicular L305 L306
  constraint perpendicular L304 L307
  constraint perpendicular L307 L308
  constraint perpendicular L309 L310
  constraint perpendicular L307 L311
  constraint perpendicular L304 L312
  constraint horizontal L313
  constraint vertical L314
  constraint horizontal L315
  constraint vertical L316
  constraint coincident L313.start L316.end
  constraint coincident L316 L317.end
  constraint coincident L316 L318.end
  constraint perpendicular L316 L319
  constraint perpendicular L319 L320
  constraint perpendicular L316 L321
  constraint perpendicular L321 L322
  constraint perpendicular L322 L323
  constraint perpendicular L323 L324
  constraint perpendicular L324 L325
  constraint perpendicular L323 L326
  constraint coincident L313 L327.end
  constraint perpendicular L326 L327
  constraint perpendicular L328 L329
  constraint perpendicular L329 L330
  constraint perpendicular L330 L331
  constraint perpendicular L329 L332
  constraint perpendicular L332 L333
  constraint perpendicular L333 L334
  constraint perpendicular L313 L335
  constraint perpendicular L316 L336
  constraint perpendicular L336 L337
  constraint perpendicular L337 L338
  constraint perpendicular L338 L339
  constraint perpendicular L337 L340
  constraint perpendicular L340 L341
  constraint perpendicular L341 L342
  constraint perpendicular L342 L343
  constraint perpendicular L341 L344
  constraint perpendicular L319 L345
  constraint perpendicular L345 L346
  constraint perpendicular L319 L347
  constraint perpendicular L347 L348
  constraint perpendicular L348 L349
  constraint perpendicular L349 L350
  constraint perpendicular L350 L351
  constraint perpendicular L349 L352
  constraint perpendicular L352 L353
  constraint perpendicular L349 L354
  constraint perpendicular L319 L355
  constraint perpendicular L316 L356
  constraint perpendicular L319 L357
  constraint perpendicular L316 L358
  constraint perpendicular L319 L359
  constraint perpendicular L316 L360
  constraint perpendicular L319 L361
  constraint perpendicular L316 L362
  constraint perpendicular L319 L363
  constraint coincident L316 L364.end
  constraint perpendicular L316 L364
  constraint perpendicular L319 L365
  constraint perpendicular L316 L366
  constraint perpendicular L319 L367
  constraint perpendicular L316 L368
  constraint perpendicular L319 L369
  constraint perpendicular L316 L370
  constraint perpendicular L319 L371
  constraint perpendicular L316 L372
  constraint perpendicular L372 L373
  constraint perpendicular L316 L374
  constraint perpendicular L372 L375
  constraint perpendicular L316 L376
  constraint perpendicular L372 L377
  constraint perpendicular L316 L378
  constraint perpendicular L372 L379
  constraint perpendicular L316 L380
  constraint perpendicular L372 L381
  constraint perpendicular L316 L382
  constraint perpendicular L372 L383
  constraint perpendicular L316 L384
  constraint perpendicular L372 L385
  constraint perpendicular L316 L386
  constraint perpendicular L372 L387
  constraint perpendicular L316 L388
  constraint perpendicular L372 L389
  constraint perpendicular L316 L390
  constraint perpendicular L372 L391
  constraint perpendicular L316 L392
  constraint perpendicular L372 L393
  constraint perpendicular L316 L394
  constraint perpendicular L372 L395
  constraint perpendicular L316 L396
  constraint perpendicular L372 L397
  constraint perpendicular L316 L398
  constraint perpendicular L372 L399
  constraint perpendicular L316 L400
  constraint perpendicular L372 L401
  constraint perpendicular L316 L402
  constraint perpendicular L372 L403
  constraint perpendicular L316 L404
  constraint perpendicular L372 L405
  constraint perpendicular L316 L406
  constraint perpendicular L372 L407
  constraint perpendicular L316 L408
  constraint perpendicular L372 L409
  constraint perpendicular L365 L410
  constraint coincident L313 L411.end
  constraint coincident L313 L412.end
  constraint perpendicular L354 L413
  constraint perpendicular L413 L414
  constraint perpendicular L414 L415
  constraint perpendicular L413 L416
  constraint perpendicular L414 L417
  constraint perpendicular L413 L418
  constraint perpendicular L414 L419
  constraint perpendicular L413 L420
  constraint perpendicular L414 L421
  constraint perpendicular L413 L422
  constraint perpendicular L384 L423
  constraint perpendicular L413 L424
  constraint perpendicular L384 L425
  constraint perpendicular L413 L426
  constraint perpendicular L384 L427
  constraint perpendicular L413 L428
  constraint perpendicular L384 L429
  constraint perpendicular L413 L430
  constraint coincident L313 L431.end
  constraint perpendicular L313 L431
  constraint vertical L432
  constraint perpendicular L432 L433
  constraint perpendicular L433 L434
  constraint perpendicular L434 L435
  constraint perpendicular L435 L436
  constraint perpendicular L436 L437
  constraint perpendicular L437 L438
  constraint perpendicular L438 L439
  constraint perpendicular L439 L440
  constraint perpendicular L438 L441
  constraint perpendicular L441 L442
  constraint perpendicular L442 L443
  constraint perpendicular L443 L444
  constraint perpendicular L444 L445
  constraint perpendicular L445 L446
  constraint perpendicular L444 L447
  constraint perpendicular L445 L448
  constraint perpendicular L448 L449
  constraint perpendicular L432 L450
  constraint horizontal L451
  constraint perpendicular L451 L452
  constraint coincident L313 L453.start
  constraint perpendicular L313 L453
  constraint coincident L313 L455.end
  constraint perpendicular L313 L455
  constraint horizontal L456
  constraint parallel L456 L457
  constraint perpendicular L458 L459
  constraint perpendicular L451 L460
  constraint perpendicular L460 L461
  constraint perpendicular L461 L462
  constraint perpendicular L462 L463
  constraint perpendicular L463 L464
  constraint perpendicular L462 L465
  constraint perpendicular L465 L466
  constraint perpendicular L462 L467
  constraint perpendicular L465 L468
  constraint perpendicular L462 L469
  constraint perpendicular L469 L470
  constraint perpendicular L470 L471
  constraint perpendicular L471 L472
  constraint coincident L313 L473.end
  constraint perpendicular L450 L474
  constraint perpendicular L474 L475
  constraint perpendicular L475 L476
  constraint perpendicular L474 L477
  constraint perpendicular L477 L478
  constraint perpendicular L474 L479
  constraint perpendicular L479 L480
  constraint perpendicular L474 L481
  constraint perpendicular L479 L482
  constraint perpendicular L452 L483
  constraint perpendicular L451 L484
  constraint perpendicular L452 L485
  constraint perpendicular L451 L486
  constraint perpendicular L452 L487
  constraint perpendicular L451 L488
  constraint perpendicular L452 L489
  constraint perpendicular L451 L490
  constraint perpendicular L452 L491
  constraint perpendicular L451 L492
  constraint perpendicular L452 L493
  constraint perpendicular L451 L494
  constraint perpendicular L452 L495
  constraint perpendicular L495 L496
  constraint perpendicular L496 L497
  constraint perpendicular L495 L498
  constraint perpendicular L476 L499
  constraint coincident L313 L500.end
  constraint perpendicular L313 L500
  constraint perpendicular L313 L501
  constraint perpendicular L500 L502
  constraint perpendicular L313 L503
  constraint perpendicular L500 L504
  constraint perpendicular L313 L505
  constraint perpendicular L500 L506
  constraint perpendicular L313 L507
  constraint perpendicular L500 L508
  constraint perpendicular L313 L509
  constraint perpendicular L500 L510
  constraint perpendicular L313 L511
  constraint perpendicular L500 L512
  constraint perpendicular L313 L513
  constraint perpendicular L513 L514
  constraint perpendicular L514 L515
  constraint perpendicular L513 L516
  constraint perpendicular L516 L517
  constraint perpendicular L513 L518
  constraint perpendicular L518 L519
  constraint perpendicular L513 L520
  constraint perpendicular L520 L521
  constraint perpendicular L513 L522
  constraint perpendicular L522 L523
  constraint perpendicular L523 L524
  constraint perpendicular L524 L525
  constraint perpendicular L523 L526
  constraint perpendicular L526 L527
  constraint perpendicular L523 L528
  constraint perpendicular L528 L529
  constraint perpendicular L523 L530
  constraint perpendicular L530 L531
  constraint perpendicular L474 L532
  constraint perpendicular L313 L533
  constraint perpendicular L474 L534
  constraint perpendicular L313 L535
  constraint perpendicular L474 L536
  constraint perpendicular L313 L537
  constraint perpendicular L474 L538
  constraint perpendicular L313 L539
  constraint perpendicular L474 L540
  constraint perpendicular L313 L541
  constraint perpendicular L474 L542
  constraint perpendicular L313 L543
  constraint perpendicular L474 L544
  constraint perpendicular L313 L545
  constraint perpendicular L545 L546
  constraint perpendicular L546 L547
  constraint perpendicular L545 L548
  constraint perpendicular L548 L549
  constraint perpendicular L545 L550
  constraint perpendicular L550 L551
  constraint perpendicular L545 L552
  constraint perpendicular L552 L553
  constraint perpendicular L545 L554
  constraint perpendicular L554 L555
  constraint perpendicular L555 L556
  constraint coincident L313 L557.start
  constraint perpendicular L313 L557
  constraint perpendicular L557 L558
  constraint perpendicular L313 L559
  constraint perpendicular L559 L560
  constraint perpendicular L560 L561
  constraint perpendicular L561 L562
  constraint perpendicular L560 L563
  constraint perpendicular L563 L564
  constraint perpendicular L560 L565
  constraint perpendicular L565 L566
  constraint perpendicular L560 L567
  constraint perpendicular L567 L568
  constraint perpendicular L560 L569
  constraint perpendicular L569 L570
  constraint coincident L313 L571.end
  constraint perpendicular L313 L571
  constraint coincident L313 L572.end
  constraint perpendicular L572 L573
  constraint perpendicular L500 L574
  constraint perpendicular L572 L575
  constraint perpendicular L500 L576
  constraint perpendicular L572 L577
  constraint perpendicular L577 L578
  constraint perpendicular L572 L579
  constraint perpendicular L577 L580
  constraint perpendicular L572 L581
  constraint perpendicular L581 L582
  constraint coincident L313 L583.end
  constraint perpendicular L313 L583
  constraint vertical L584
  constraint perpendicular L584 L585
  constraint perpendicular L585 L586
  constraint perpendicular L586 L587
  constraint perpendicular L587 L588
  constraint perpendicular L588 L589
  constraint perpendicular L587 L590
  constraint perpendicular L590 L591
  constraint perpendicular L587 L592
  constraint perpendicular L592 L593
  constraint perpendicular L587 L594
  constraint perpendicular L584 L595
  constraint coincident L313 L596.end
  constraint perpendicular L313 L597
  constraint perpendicular L597 L598
  constraint perpendicular L596 L599
  constraint perpendicular L599 L600
  constraint perpendicular L598 L601
  constraint perpendicular L599 L602
  constraint perpendicular L602 L603
  constraint perpendicular L603 L604
  constraint perpendicular L602 L605
  constraint perpendicular L605 L606
  constraint perpendicular L602 L607
  constraint perpendicular L607 L608
  constraint perpendicular L602 L609
  constraint perpendicular L609 L610
  constraint perpendicular L608 L611
  constraint perpendicular L583 L612
  constraint perpendicular L608 L613
  constraint perpendicular L613 L614
  constraint perpendicular L608 L615
  constraint perpendicular L613 L616
  constraint perpendicular L608 L617
  constraint perpendicular L618 L619
  constraint perpendicular L618 L620
  constraint perpendicular L620 L621
  constraint perpendicular L621 L622
  constraint perpendicular L604 L623
  constraint perpendicular L623 L624
  constraint perpendicular L624 L625
  constraint perpendicular L623 L626
  constraint perpendicular L624 L627
  constraint perpendicular L623 L628
  constraint perpendicular L624 L629
  constraint perpendicular L623 L630
  constraint perpendicular L624 L631
  constraint perpendicular L623 L632
  constraint perpendicular L624 L633
  constraint perpendicular L623 L634
  constraint perpendicular L624 L635
  constraint perpendicular L623 L636
  constraint perpendicular L624 L637
  constraint perpendicular L623 L638
  constraint coincident L313 L639.end
  constraint perpendicular L313 L639
  constraint perpendicular L594 L640
  constraint perpendicular L313 L641
  constraint perpendicular L594 L642
  constraint perpendicular L313 L643
  constraint perpendicular L594 L644
  constraint perpendicular L313 L645
  constraint perpendicular L594 L646
  constraint perpendicular L313 L647
  constraint perpendicular L594 L648
  constraint perpendicular L313 L649
  constraint perpendicular L594 L650
  constraint perpendicular L313 L651
  constraint perpendicular L594 L652
  constraint perpendicular L313 L653
  constraint perpendicular L594 L654
  constraint perpendicular L654 L655
  constraint perpendicular L605 L656
  constraint perpendicular L606 L657
  constraint perpendicular L605 L658
  constraint perpendicular L606 L659
  constraint perpendicular L605 L660
  constraint perpendicular L661 L662
  constraint perpendicular L663 L664
  constraint perpendicular L660 L668
  constraint perpendicular L661 L669
  constraint perpendicular L665 L670
  constraint perpendicular L670 L671
  constraint perpendicular L665 L672
  constraint perpendicular L672 L673
  constraint perpendicular L665 L674
  constraint perpendicular L674 L675
  constraint perpendicular L665 L676
  constraint perpendicular L313 L677
  constraint perpendicular L665 L678
  constraint perpendicular L313 L679
  constraint perpendicular L665 L680
  constraint perpendicular L313 L681
  constraint perpendicular L665 L682
  constraint perpendicular L313 L683
  constraint perpendicular L665 L684
  constraint perpendicular L313 L685
  constraint perpendicular L665 L686
  constraint perpendicular L686 L687
  constraint perpendicular L687 L688
  constraint perpendicular L686 L689
  constraint perpendicular L689 L690
  constraint perpendicular L640 L691
  constraint vertical L692
  constraint perpendicular L692 L693
  constraint perpendicular L693 L694
  constraint perpendicular L692 L695
  constraint perpendicular L695 L696
  constraint perpendicular L692 L697
  constraint horizontal L698
  constraint vertical L699
  constraint horizontal L700
  constraint vertical L701
  constraint perpendicular L697 L702
  constraint perpendicular L692 L703
  measures "d3" distance of L0.start L0.end
  measures "d4" distance of L0.end L1.end
  measures "d5" distance of L1.end L2.end
  measures "d6" distance of L2.end L3.end
  measures "d7" distance of L3.end L4.end
  measures "d8" distance of L4.end L5.end
  measures "d9" distance of L5.end L6.end
  measures "d10" distance of L6.end L7.end
  measures "d11" distance of L8.end L9.end
  measures "d12" distance of L9.end L10.end
  measures "d13" distance of L10.end L11.end
  measures "d14" distance of L12.end L14.end
  measures "d18" distance of L10.end L15.start
  measures "d19" distance of L16.end L17.end
  measures "d20" distance of L14.end L18.end
  measures "d21" distance of L18.end L19.end
  measures "d22" distance of L19.end L20.end
  measures "d23" distance of L17.end L22.end
  measures "d24" distance of L211.end L271.end